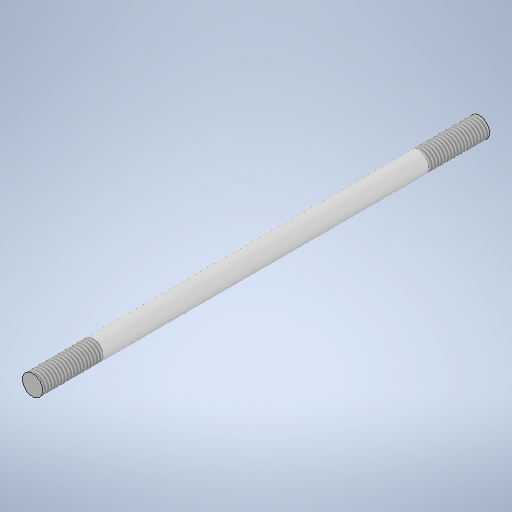
# Autodesk Inventor part: TS_V1_Fallmagazin_Verbindungsstange_int
Saved by Autodesk Inventor 2025.2 (Build 292293000, 293)
## iProperties
Created: 2025-06-19
Part Number: TS_V1_Fallmagazin_Verbindungsstange_int
Material: Generisch
Document SubType Name: Modeling
Designer: tino
Density: 1 g/cm^3
Appearance: Vorgabe
Author: tino
Autodesk Inventor part; units mm, degrees
ref_plane "YZ Plane" through (0, 0, 0) normal (1, 0, 0) x (0, 1, 0)
ref_plane "XZ Plane" through (0, 0, 0) normal (0, 1, 0) x (-1, 0, 0)
ref_plane "XY Plane" through (0, 0, 0) normal (0, 0, 1) x (1, 0, 0)
sketch "Skizze1" plane through (0, 0, 0) normal (1, 0, 0) x (0, 1, 0)
  line L0 (-55, 2.5) -> (0, 2.5)
  line L1 (0, 2.5) -> (0, 0)
  line L2 (0, 0) -> (-55, 0)
  line L3 (-55, 0) -> (-55, 2.5)
  point P0 (-55, 1.25)
  dimension "d2" = 55
  dimension "d3" = 2.5
  constraints: 8 end point, 2 parallel, 2 point on line, 1 horizontal, 1 midpoint, 1 perpendicular
  measures "d2" distance of L0.start L0.end
  measures "d3" distance of L2.end L0.start
revolve "Umdrehung1" add sketch "Skizze1" angle 360 about axis through (0, 0, 0) along (0, -1, 0)
thread "Gewinde1" size "M5x0.8" class "6g" standard "ANSI Metric M Profile" length 15 offset 40
mirror "Spiegeln1" about plane through (0, 0, 2.5) normal (0, 1, 0) of "Umdrehung1"
thread "Gewinde2" size "M5x0.8" class "6g" standard "ANSI Metric M Profile" length 15
